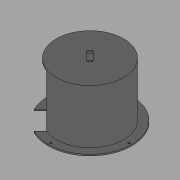
# Autodesk Inventor part: mechanism_cover
Saved by Autodesk Inventor 2019 (Build 230136000, 136)
## iProperties
Part Number: mechanism_cover
Material: Generic
Document SubType Name: Modeling
Designer: Javi
Appearance: Default
Author: Javi
Autodesk Inventor part; units mm, degrees
ref_plane "XZ Plane" through (0, 0, 0) normal (0, 1, 0) x (-1, 0, 0)
ref_plane "XY Plane" through (0, 0, 0) normal (0, 0, 1) x (1, 0, 0)
sketch "Sketch1" plane through (0, 0, 0) normal (0, 1, 0) x (-1, 0, 0)
  circle A0 centre (0, 0) radius 120
  circle A1 centre (0, 0) radius 125
  circle A2 centre (0, 0) radius 155
  dimension "d0" = 240
  dimension "d1" = 250
  dimension "d2" = 310
  constraints: 3 centre point, 3 coincident
  measures "d0" diameter of A0
  measures "d1" diameter of A1
  measures "d2" diameter of A2
extrude "Extrusion1" add sketch "Sketch1" along normal blind 205 contours A0 | A1 | A2
sketch "Sketch3" plane through (0, 205, 0) normal (0, 1, 0) x (1, 0, 0)
  circle A0 centre (0, 0) radius 155
  circle A1 centre (0, 0) radius 125
  dimension "d27" = 250
  dimension "d28" = 310
  constraints: 2 centre point, 2 coincident
  measures "d27" diameter of A1
  measures "d28" diameter of A0
extrude "Extrusion3" cut sketch "Sketch3" against normal blind 200
sketch "Sketch4" plane through (0, 5, 0) normal (0, 1, 0) x (1, 0, 0)
  circle A0 centre (0, 145) radius 4.5
  circle A1 centre (0, 0) radius 155 projected
  line L0 (0, 155) -> (0, 125)
  circle A2 centre (0, 0) radius 125 projected
  circle A3 centre (-145, 0) radius 4.5
  line L1 (-155, 0) -> (-125, 0)
  circle A4 centre (0, -145) radius 4.5
  line L2 (0, -155) -> (0, -125)
  circle A5 centre (145, 0) radius 4.5
  line L3 (155, 0) -> (125, 0)
  dimension "d31" = 9
  dimension "d32" = 0
  dimension "d33" = 145
  dimension "d36" = 360
  constraints: 8 end point, 4 centre point, 2 vertical, 2 vertical alignment, 23 other
  measures "d31" diameter of A0
  measures "d32" distance from line of L0 A0.centre
  measures "d33" distance of point (0, 0) A0.centre
extrude "Extrusion4" cut sketch "Sketch4" against normal through all contours A0 L0 | L0 A0 | L3 A5 | A5 L3 | L1 A3 | A3 L1 | L2 A4 | A4 L2
sketch "Sketch5" plane through (0, 0, 0) normal (0, -1, 0) x (1, 0, 0)
  circle A0 centre (0, 0) radius 120
  dimension "d40" = 240
  constraints: 1 centre point, 1 coincident
  measures "d40" diameter of A0
extrude "Extrusion5" cut sketch "Sketch5" against normal blind 200
ref_plane "Work Plane2" through (-109.6016, 0, 109.6016) normal (0.7071068, 0, -0.7071068) x (0, 1, 0)
ref_plane "Work Plane1" through (0, 0, 0) normal (0.7071068, 0, -0.7071068) x (0, 1, 0)
sketch "Sketch6" plane through (-109.6016, 0, 109.6016) normal (0.7071068, 0, -0.7071068) x (0, 1, 0)
  line L0 (0, -50) -> (200, -50)
  line L1 (200, -50) -> (200, 50)
  line L2 (200, 50) -> (0, 50)
  line L3 (0, 50) -> (0, -50)
  line L4 (0, 155) -> (0, -155) projected
  line L5 (-41, 0) -> (246, 0) projected
  point P0 (0, 0)
  dimension "d44" = 200
  dimension "d45" = 100
  dimension "d46" = 0
  dimension "d47" = 50
  constraints: 8 end point, 2 parallel, 1 horizontal, 1 perpendicular
  measures "d44" distance of L2.end L1.end
  measures "d45" distance of L1.end L0.end
  measures "d46" distance between parallel lines of L4 L3
  measures "d47" distance between parallel lines of L5 L0
extrude "Extrusion6" cut sketch "Sketch6" along normal up to surface round surface about axis through (0, 0, 0) along (0, 1, 0) radius 120 far side no
sketch "Sketch7" plane through (0, 205, 0) normal (0, 1, 0) x (1, 0, 0)
  circle A0 centre (0, 0) radius 10
  line L0 (0, 0) -> (31, 0) construction
  line L1 (7.0711, 7.0711) -> (-14.2128, 28.355)
  line L2 (-14.2128, 28.355) -> (-28.355, 14.2128)
  line L3 (-28.355, 14.2128) -> (-7.0711, -7.0711)
  line L4 (-7.0711, -7.0711) -> (0.2828, -14.425)
  line L5 (-7.0711, -7.0711) -> (3.3289, -7.0711) construction
  line L6 (0.2828, -14.425) -> (14.425, -0.2828)
  line L7 (14.425, -0.2828) -> (7.0711, 7.0711)
  circle A1 centre (-28.0368, 20.9657) radius 1.75
  circle A2 centre (-20.9657, 28.0368) radius 1.75
  circle A3 centre (7.6721, -14.7432) radius 1.75
  circle A4 centre (14.7432, -7.6721) radius 1.75
  dimension "d50" = 20
  dimension "d53" = 20
  dimension "d55" = 10.4
  dimension "d56" = 45
  dimension "d57" = 30.1
  dimension "d58" = 3.5
  dimension "d61" = 5
  dimension "d65" = 10
  dimension "d68" = 50.5
  dimension "d71" = 4.55
  constraints: 16 end point, 5 centre point, 3 perpendicular, 3 tangent, 2 horizontal, 2 point on circle, 1 coincident, 1 equal length, 1 point on line, 8 other
  measures "d50" diameter of A0
  measures "d53" distance of L1.end L2.end
  measures "d55" distance of L3.end L4.end
  measures "d56" angle of L4 L5
  measures "d57" distance from line of L3.end L2
  measures "d58" diameter of A1
  measures "d61" distance from line of L3 A1.centre
  measures "d65" distance of A1.centre A2.centre
  measures "d68" distance of A1.centre A3.centre
  measures "d71" distance from line of L2 A2.centre
extrude "Extrusion7" cut sketch "Sketch7" against normal through all
body "Solid1"
